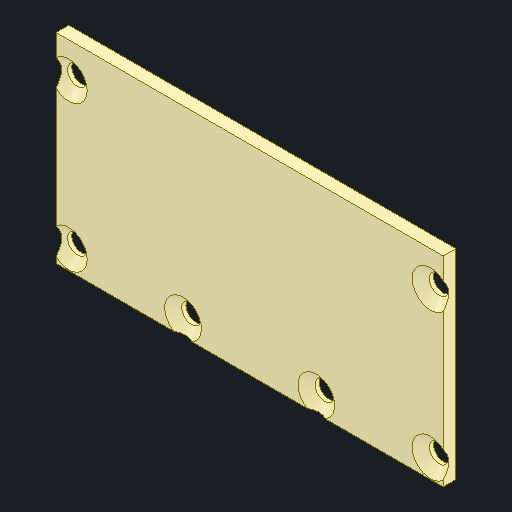
# Autodesk Inventor part: back
Saved by Autodesk Inventor 2023 (Build 270158000, 158)
## iProperties
Created: 2024-05-19
Part Number: back
Material: Nylon 6/6
Document SubType Name: Modeling
Designer: szymo
Density: 1.13 g/cm^3
Appearance: Nylon 6
Mass: 3.55716 g
Surface Area: 44.8969 cm^2
Volume: 3.14793 cm^3
Author: szymo
Autodesk Inventor part; units mm, degrees
ref_plane "YZ Plane" through (0, 0, 0) normal (1, 0, 0) x (0, 1, 0)
ref_plane "XZ Plane" through (0, 0, 0) normal (0, 1, 0) x (-1, 0, 0)
ref_plane "XY Plane" through (0, 0, 0) normal (0, 0, 1) x (1, 0, 0)
ref_plane "Work Plane1" through (22, 31.5, 0) normal (0, 0, 1) x (0, 1, 0)
sketch "Sketch1" plane through (22, 31.5, 0) normal (0, 0, 1) x (0, 1, 0)
  line L0 (0, 0) -> (0, 61) projected
  line L1 (0, 61) -> (-3.5, 61) projected
  line L2 (-3.5, 0) -> (-3.5, 61) projected
  circle A0 centre (-5.5, 2) radius 1.75 projected
  circle A1 centre (-28.5, 2) radius 1.75 projected
  line L3 (-3.5, 4) -> (-7.5, 4) projected
  arc A2 (-8.5, 3) -> (-7.5, 4) centre (-8.5, 4) ccw projected
  line L4 (-8.5, 3) -> (-21.7679, 3) projected
  arc A3 (-23.5, 4) -> (-21.7679, 3) centre (-21.7679, 5) ccw projected
  line L5 (-23.5, 4) -> (-31.5, 4) projected
  line L6 (-31.5, 0) -> (-31.5, 4) projected
  line L7 (-3.5, 0) -> (-3.5, 4) projected
  line L8 (-23.5, 22) -> (-3.5, 22) projected
  line L9 (-3.5, 22) -> (-3.5, 18) projected
  line L10 (-23.5, 39) -> (-3.5, 39) projected
  line L11 (-3.5, 39) -> (-3.5, 43) projected
  line L12 (-3.5, 57) -> (-6.7679, 57) projected
  line L13 (-3.5, 61) -> (-3.5, 57) projected
  line L14 (-3.5, 61) -> (-31.5, 61) projected
  line L15 (-31.5, 61) -> (-31.5, 57) projected
  line L16 (-24.004, 57) -> (-31.5, 57) projected
  line L17 (0, 0) -> (-31.5, 0)
  line L18 (-31.5, 0) -> (-31.5, 61)
  line L19 (-31.5, 61) -> (0, 61)
  line L20 (0, 61) -> (0, 0)
  line L21 (-3.5, 0) -> (-31.5, 0)
  line L22 (-8.5, 58) -> (-21.7679, 58) projected
  arc A4 (-7.634, 57.5) -> (-6.7679, 57) centre (-6.7679, 58) ccw projected
  arc A5 (-24.004, 57) -> (-23.2587, 57.3333) centre (-24.004, 58) ccw projected
  arc A6 (-21.7679, 58) -> (-23.2587, 57.3333) centre (-21.7679, 56) ccw projected
  arc A7 (-7.634, 57.5) -> (-8.5, 58) centre (-8.5, 57) ccw projected
  circle A8 centre (-5.5, 59) radius 1.75 projected
  circle A9 centre (-28.5, 59) radius 1.75 projected
  line L23 (-23.5, 18) -> (-23.5, 22) projected
  line L24 (-23.5, 18) -> (-3.5, 18) projected
  line L25 (-23.5, 43) -> (-3.5, 43) projected
  line L26 (-23.5, 43) -> (-23.5, 39) projected
  point P0 (-3.5, 28.5)
  point P1 (-3.5, 32.5)
  point P2 (-3.5, 61)
  point P3 (-13.5, 58)
  dimension "d25" = 0
  dimension "d26" = 0
  constraints: 10 end point, 1 horizontal, 1 parallel, 1 perpendicular, 1 vertical, 1 other
  measures "d25" distance between parallel lines of L19 L1
  measures "d26" distance from line of point (-3.5, 0) L17
extrude "Extrusion1" add sketch "Sketch1" along normal blind 2 contours L17 L2 L1 L0 | L17 L6 L5 A3 L4 A2 L3 L2 | L2 L12 A4 A7 L22 A6 A5 L16 L15 L14 | L3 A2 L4 A3 L5 L18 L16 A5 A6 L22 A7 A4 L12 L2 L25 L26 L10 L8 L23 L24 | L24 L23 L8 L2 | L2 L10 L26 L25 | A0 | A1 | A8 | A9
sketch "Sketch2" plane through (22, 31.5, 2) normal (0, 0, 1) x (1, 0, 0)
  circle A0 centre (-2, -5.5) radius 1.75 projected
  circle A1 centre (-2, -28.5) radius 1.75 projected
  arc A2 (-4, -6.7679) -> (-3.5, -7.634) centre (-3, -6.7679) ccw projected
  arc A3 (-3, -8.5) -> (-3.5, -7.634) centre (-4, -8.5) ccw projected
  line L0 (-3, -8.5) -> (-3, -21.7679) projected
  arc A4 (-3.6667, -23.2587) -> (-3, -21.7679) centre (-5, -21.7679) ccw projected
  arc A5 (-3.6667, -23.2587) -> (-4, -24.004) centre (-3, -24.004) ccw projected
  line L1 (-4, -24.004) -> (-4, -31.5) projected
  line L2 (0, -31.5) -> (-4, -31.5) projected
  line L3 (0, -3.5) -> (0, -31.5) projected
  line L4 (0, -3.5) -> (-4, -3.5) projected
  line L5 (-4, -3.5) -> (-4, -6.7679) projected
  line L6 (-39, -23.5) -> (-39, -3.5) projected
  line L7 (-39, -3.5) -> (-43, -3.5) projected
  line L8 (-43, -23.5) -> (-43, -3.5) projected
  line L9 (-43, -23.5) -> (-39, -23.5) projected
  circle A6 centre (-59, -5.5) radius 1.75 projected
  circle A7 centre (-59, -28.5) radius 1.75 projected
  arc A8 (-57.5, -7.634) -> (-57, -6.7679) centre (-58, -6.7679) ccw projected
  line L10 (-57, -3.5) -> (-57, -6.7679) projected
  line L11 (-61, -3.5) -> (-57, -3.5) projected
  line L12 (-61, -3.5) -> (-61, -31.5) projected
  line L13 (-61, -31.5) -> (-57, -31.5) projected
  line L14 (-57, -24.004) -> (-57, -31.5) projected
  arc A9 (-57, -24.004) -> (-57.3333, -23.2587) centre (-58, -24.004) ccw projected
  arc A10 (-58, -21.7679) -> (-57.3333, -23.2587) centre (-56, -21.7679) ccw projected
  line L15 (-58, -8.5) -> (-58, -21.7679) projected
  arc A11 (-57.5, -7.634) -> (-58, -8.5) centre (-57, -8.5) ccw projected
  line L16 (-22, -23.5) -> (-22, -3.5) projected
  line L17 (-18, -23.5) -> (-22, -23.5) projected
  line L18 (-18, -23.5) -> (-18, -3.5) projected
  line L19 (-22, -3.5) -> (-18, -3.5) projected
  circle A12 centre (-20, -29) radius 1.75 projected
  line L20 (-22, -31.5) -> (-18, -31.5) projected
  line L21 (-18, -31.5) -> (-18, -23.5) projected
  line L22 (-22, -23.5) -> (-18, -23.5) projected
  line L23 (-22, -23.5) -> (-22, -31.5) projected
  circle A13 centre (-41, -29) radius 1.75 projected
  line L24 (-39, -31.5) -> (-43, -31.5) projected
  line L25 (-39, -23.5) -> (-39, -31.5) projected
  line L26 (-39, -23.5) -> (-43, -23.5) projected
  line L27 (-43, -31.5) -> (-43, -23.5) projected
  constraints: 4 coincident
hole "Hole1" at (20, 3, 2) at (20, 26, 2) at (2, 2.5, 2) at (-19, 2.5, 2) at (-37, 26, 2) at (-37, 3, 2) direction (0, 0, -1) diameter 3.1 end through all countersink diameter 5.8 countersink angle 90 clearance for "Countersunk Flat Head Screw ISO 2009/7046" size "M2.5" standard "ISO"
sketch "Sketch4" plane through (22, 31.5, 0) normal (0, 0, -1) x (-1, 0, 0)
  circle A0 centre (2, -5.5) radius 1.75
  circle A1 centre (2, -28.5) radius 1.75
  arc A2 (3.5, -7.634) -> (4, -6.7679) centre (3, -6.7679) ccw
  arc A3 (3.5, -7.634) -> (3, -8.5) centre (4, -8.5) ccw
  line L0 (3, -8.5) -> (3, -21.7679)
  arc A4 (3, -21.7679) -> (3.6667, -23.2587) centre (5, -21.7679) ccw
  arc A5 (4, -24.004) -> (3.6667, -23.2587) centre (3, -24.004) ccw
  line L1 (4, -24.004) -> (4, -31.5)
  line L2 (0, -31.5) -> (4, -31.5)
  line L3 (0, -3.5) -> (0, -31.5)
  line L4 (0, -3.5) -> (4, -3.5)
  line L5 (4, -3.5) -> (4, -6.7679)
  line L6 (39, -23.5) -> (39, -3.5)
  line L7 (39, -3.5) -> (43, -3.5)
  line L8 (43, -23.5) -> (43, -3.5)
  line L9 (43, -23.5) -> (39, -23.5)
  line L10 (22, -23.5) -> (22, -3.5)
  line L11 (18, -23.5) -> (22, -23.5)
  line L12 (18, -23.5) -> (18, -3.5)
  line L13 (22, -3.5) -> (18, -3.5)
  circle A6 centre (20, -29) radius 1.75
  line L14 (22, -31.5) -> (18, -31.5)
  line L15 (18, -31.5) -> (18, -23.5)
  line L16 (22, -23.5) -> (18, -23.5)
  line L17 (22, -23.5) -> (22, -31.5)
  circle A7 centre (41, -29) radius 1.75
  line L18 (39, -31.5) -> (43, -31.5)
  line L19 (39, -23.5) -> (39, -31.5)
  line L20 (39, -23.5) -> (43, -23.5)
  line L21 (43, -31.5) -> (43, -23.5)
  circle A8 centre (59, -5.5) radius 1.75
  circle A9 centre (59, -28.5) radius 1.75
  arc A10 (57, -6.7679) -> (57.5, -7.634) centre (58, -6.7679) ccw
  line L22 (57, -3.5) -> (57, -6.7679)
  line L23 (61, -3.5) -> (57, -3.5)
  line L24 (61, -3.5) -> (61, -31.5)
  line L25 (61, -31.5) -> (57, -31.5)
  line L26 (57, -24.004) -> (57, -31.5)
  arc A11 (57.3333, -23.2587) -> (57, -24.004) centre (58, -24.004) ccw
  arc A12 (57.3333, -23.2587) -> (58, -21.7679) centre (56, -21.7679) ccw
  line L27 (58, -8.5) -> (58, -21.7679)
  arc A13 (58, -8.5) -> (57.5, -7.634) centre (57, -8.5) ccw
  line L28 (61, -31.5) -> (42.4697, -31.5)
  line L29 (0, -31.5) -> (0, 0)
  line L30 (61, -31.5) -> (0, -31.5)
  line L31 (0, -31.5) -> (0, -25.5)
  line L32 (0, -25.5) -> (61, -25.5)
  line L33 (61, -25.5) -> (61, -31.5)
  line L34 (61, 0) -> (61, -31.5)
  line L35 (0, -8.5) -> (61, -8.5)
  line L36 (61, -8.5) -> (61, -2.5)
  line L37 (61, -2.5) -> (0, -2.5)
  line L38 (0, -2.5) -> (0, -8.5)
  circle A14 centre (41, -29) radius 1.55
  line L39 (59, -5.5) -> (41, -29) construction
  line L40 (2, -5.5) -> (20, -29) construction
  arc A15 (42.4697, -31.5) -> (39.5303, -31.5) centre (41, -29) ccw
  line L41 (41, -29) -> (30.5, -8.5) construction
  line L42 (20, -29) -> (30.5, -8.5) construction
  circle A16 centre (2, -28.5) radius 1.55
  line L43 (57, -25.5) -> (57, -8.5)
  line L44 (4, -25.5) -> (4, -8.5)
  line L45 (57, -10.5779) -> (45.5703, -25.5)
  line L46 (54.8127, -8.5) -> (41.7914, -25.5)
  line L47 (40.8926, -25.5) -> (32.1853, -8.5)
  line L48 (28.8147, -8.5) -> (20.1817, -25.3548)
  line L49 (23.478, -25.5) -> (30.5, -11.7904)
  line L50 (30.5, -11.7904) -> (37.522, -25.5)
  line L51 (19.2086, -25.5) -> (6.1873, -8.5)
  line L52 (4, -10.5779) -> (15.4297, -25.5)
  arc A17 (21.4697, -31.5) -> (18.5303, -31.5) centre (20, -29) ccw
  line L53 (18.5303, -31.5) -> (0, -31.5)
  line L54 (0, -31.5) -> (0, -30.6)
  line L55 (0, 0) -> (61, 0)
  line L56 (61, 0) -> (61, -3.4)
  line L57 (61, -31.5) -> (42.4697, -31.5)
  arc A18 (42.4697, -31.5) -> (39.5303, -31.5) centre (41, -29) ccw
  line L58 (39.5303, -31.5) -> (21.4697, -31.5)
  arc A19 (61, -26.4) -> (61, -30.6) centre (59, -28.5) ccw
  arc A20 (0, -7.6) -> (0, -3.4) centre (2, -5.5) ccw
  arc A21 (0, -30.6) -> (0, -26.4) centre (2, -28.5) ccw
  arc A22 (61, -3.4) -> (61, -7.6) centre (59, -5.5) ccw
  line L59 (61, -7.6) -> (61, -26.4)
  line L60 (61, -30.6) -> (61, -31.5)
  line L61 (0, -26.4) -> (0, -7.6)
  line L62 (0, -3.4) -> (0, 0)
  point P0 (4, -24.004)
  point P1 (18, -23.9221)
  point P2 (18, -8.5)
  point P3 (22, -21.8049)
  point P4 (22, -8.5)
  point P5 (39, -21.8049)
  point P6 (39, -8.5)
  point P7 (43, -23.9221)
  point P8 (43, -8.5)
  point P9 (0, -2.5)
extrude "Extrusion3" cut sketch "Sketch4" against normal blind 1 contours L35 L12 L15 L51 | L52 L32 L1 L44 | L35 L48 L10 | L35 L6 L47 | L49 L50 L32 | L46 L21 L8 L35 | L43 L26 L32 L45
body "Solid1"
